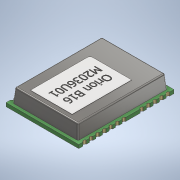
# Autodesk Inventor part: 03-0002
Saved by Autodesk Inventor 2021 (Build 250183000, 183)
## iProperties
Created: 2021-11-16
Part Number: 03-0002
Material: Stainless Steel
Document SubType Name: Modeling
Designer: Bradley
Density: 8 g/cm^3
Appearance: Semi-Polished
Author: Bradley
Autodesk Inventor part; units mm, degrees
ref_plane "YZ Plane" through (0, 0, 0) normal (1, 0, 0) x (0, 1, 0)
ref_plane "XZ Plane" through (0, 0, 0) normal (0, 1, 0) x (-1, 0, 0)
ref_plane "XY Plane" through (0, 0, 0) normal (0, 0, 1) x (1, 0, 0)
sketch "Sketch1" plane through (0, 0, 0) normal (0, 0, 1) x (1, 0, 0)
  line L0 (-6.1, -8) -> (6.1, -8)
  line L1 (6.1, -8) -> (6.1, 8)
  line L2 (6.1, 8) -> (-6.1, 8)
  line L3 (-6.1, 8) -> (-6.1, -8)
  line L4 (-6.1, -8) -> (6.1, 8) construction
  line L5 (6.1, -8) -> (-6.1, 8) construction
  point P0 (0, 0)
  dimension "d0" = 12.2
  dimension "d1" = 16
  constraints: 12 end point, 2 midpoint, 2 parallel, 1 horizontal, 1 perpendicular
  measures "d0" distance of L2.end L1.end
  measures "d1" distance of L1.end L0.end
extrude "Extrusion1" add sketch "Sketch1" along normal mid plane 0.6
sketch "Sketch2" plane through (0, 0, 0.3) normal (0, 0, 1) x (1, 0, 0)
  line L0 (6.1, -8) -> (6.1, 8) projected
  line L1 (6.1, 8) -> (-6.1, 8) projected
  line L2 (-6.1, 8) -> (-6.1, -8) projected
  line L3 (-6.1, -8) -> (6.1, -8) projected
  line L4 (-6.1, 8) -> (-6.1, -8) projected
  arc A0 (-6.1, 2.3) -> (-6.1, 2.9) centre (-6.2, 2.6) ccw
  line L5 (6.1, -8) -> (6.1, 8) projected
  arc A1 (6.1, 2.9) -> (6.1, 2.3) centre (6.2, 2.6) ccw
  arc A2 (-6.1, -7.3) -> (-6.1, -6.7) centre (-6.2, -7) ccw
  arc A3 (6.1, -6.7) -> (6.1, -7.3) centre (6.2, -7) ccw
  arc A4 (-6.1, 3.4) -> (-6.1, 4) centre (-6.2, 3.7) ccw
  arc A5 (6.1, 4) -> (6.1, 3.4) centre (6.2, 3.7) ccw
  arc A6 (-6.1, -6.2) -> (-6.1, -5.6) centre (-6.2, -5.9) ccw
  arc A7 (6.1, -5.6) -> (6.1, -6.2) centre (6.2, -5.9) ccw
  arc A8 (-6.1, 4.5) -> (-6.1, 5.1) centre (-6.2, 4.8) ccw
  arc A9 (6.1, 5.1) -> (6.1, 4.5) centre (6.2, 4.8) ccw
  arc A10 (-6.1, -5.1) -> (-6.1, -4.5) centre (-6.2, -4.8) ccw
  arc A11 (6.1, -4.5) -> (6.1, -5.1) centre (6.2, -4.8) ccw
  arc A12 (-6.1, 5.6) -> (-6.1, 6.2) centre (-6.2, 5.9) ccw
  arc A13 (6.1, 6.2) -> (6.1, 5.6) centre (6.2, 5.9) ccw
  arc A14 (-6.1, -4) -> (-6.1, -3.4) centre (-6.2, -3.7) ccw
  arc A15 (6.1, -3.4) -> (6.1, -4) centre (6.2, -3.7) ccw
  arc A16 (-6.1, 6.7) -> (-6.1, 7.3) centre (-6.2, 7) ccw
  arc A17 (6.1, 7.3) -> (6.1, 6.7) centre (6.2, 7) ccw
  arc A18 (-6.1, -2.9) -> (-6.1, -2.3) centre (-6.2, -2.6) ccw
  arc A19 (6.1, -2.3) -> (6.1, -2.9) centre (6.2, -2.6) ccw
  arc A20 (-6.1, 7.8) -> (-6.1, 8.4) centre (-6.2, 8.1) ccw
  arc A21 (6.1, 8.4) -> (6.1, 7.8) centre (6.2, 8.1) ccw
  arc A22 (-6.1, -1.8) -> (-6.1, -1.2) centre (-6.2, -1.5) ccw
  arc A23 (6.1, -1.2) -> (6.1, -1.8) centre (6.2, -1.5) ccw
  arc A24 (-6.1, 8.9) -> (-6.1, 9.5) centre (-6.2, 9.2) ccw
  arc A25 (6.1, 9.5) -> (6.1, 8.9) centre (6.2, 9.2) ccw
  arc A26 (-6.1, -0.7) -> (-6.1, -0.1) centre (-6.2, -0.4) ccw
  arc A27 (6.1, -0.1) -> (6.1, -0.7) centre (6.2, -0.4) ccw
  point P0 (0, 0)
  point P1 (-6.1, -5.1)
  point P2 (-6.1, -0.1)
  point P3 (-6.1, 2.9)
  point P4 (-6.1, 4)
  point P5 (6.1, 5.6)
  point P6 (6.1, 3.4)
  point P7 (6.1, 2.3)
  point P8 (6.1, -0.7)
  point P9 (6.1, -1.8)
  point P10 (6.1, -2.9)
  point P11 (6.1, -4)
  point P12 (6.1, -6.2)
  point P13 (6.1, -7.3)
  dimension "d4" = 1
  dimension "d5" = 0.6
  dimension "d6" = 0.1
  dimension "d7" = 0.1
  dimension "d10" = 1.1
  dimension "d15" = 3
  constraints: 74 vertical alignment, 56 point on circle, 28 centre point, 27 equal radius, 8 point on line, 2 horizontal alignment, 2 other
  measures "d4" distance from line of L3 A3.centre
  measures "d5" distance of A3.end A3.start
  measures "d10" distance of A0.start A4.start
  measures "d15" distance of A27.centre A1.centre
extrude "Extrusion2" cut sketch "Sketch2" against normal through all contours A3 L0 | L2 A2 | A7 L0 | L2 A6 | A11 L0 | L2 A10 | A15 L0 | L2 A14 | A19 L0 | L2 A18 | A23 L0 | L2 A22 | A27 L0 | L2 A26 | A1 L0 | L2 A0 | A5 L0 | L2 A4 | A9 L0 | L2 A8 | A13 L0 | L2 A12 | A17 L0 | L2 A16
sketch "Sketch3" plane through (0, 0, 0.3) normal (0, 0, 1) x (1, 0, 0)
  arc A0 (6.1, -4.5) -> (6.1, -5.1) centre (6.2, -4.8) ccw projected
  line L0 (6.1, -4.5) -> (6.1, -4) projected
  arc A1 (6.1, -3.4) -> (6.1, -4) centre (6.2, -3.7) ccw projected
  line L1 (6.1, -3.4) -> (6.1, -2.9) projected
  arc A2 (6.1, -2.3) -> (6.1, -2.9) centre (6.2, -2.6) ccw projected
  line L2 (6.1, -2.3) -> (6.1, -1.8) projected
  arc A3 (6.1, -1.2) -> (6.1, -1.8) centre (6.2, -1.5) ccw projected
  line L3 (6.1, -1.2) -> (6.1, -0.7) projected
  arc A4 (6.1, -0.1) -> (6.1, -0.7) centre (6.2, -0.4) ccw projected
  line L4 (6.1, -0.1) -> (6.1, 2.3) projected
  arc A5 (6.1, 2.9) -> (6.1, 2.3) centre (6.2, 2.6) ccw projected
  line L5 (6.1, 2.9) -> (6.1, 3.4) projected
  arc A6 (6.1, 4) -> (6.1, 3.4) centre (6.2, 3.7) ccw projected
  line L6 (6.1, 4) -> (6.1, 4.5) projected
  arc A7 (6.1, 5.1) -> (6.1, 4.5) centre (6.2, 4.8) ccw projected
  line L7 (6.1, 5.1) -> (6.1, 5.6) projected
  arc A8 (6.1, 6.2) -> (6.1, 5.6) centre (6.2, 5.9) ccw projected
  line L8 (6.1, 6.2) -> (6.1, 6.7) projected
  arc A9 (6.1, 7.3) -> (6.1, 6.7) centre (6.2, 7) ccw projected
  line L9 (6.1, 7.3) -> (6.1, 8) projected
  line L10 (6.1, 8) -> (-6.1, 8) projected
  line L11 (-6.1, 8) -> (-6.1, 7.3) projected
  arc A10 (-6.1, 6.7) -> (-6.1, 7.3) centre (-6.2, 7) ccw projected
  line L12 (-6.1, 6.7) -> (-6.1, 6.2) projected
  arc A11 (-6.1, 5.6) -> (-6.1, 6.2) centre (-6.2, 5.9) ccw projected
  line L13 (-6.1, 5.6) -> (-6.1, 5.1) projected
  arc A12 (-6.1, 4.5) -> (-6.1, 5.1) centre (-6.2, 4.8) ccw projected
  line L14 (-6.1, 4.5) -> (-6.1, 4) projected
  arc A13 (-6.1, 3.4) -> (-6.1, 4) centre (-6.2, 3.7) ccw projected
  line L15 (-6.1, 3.4) -> (-6.1, 2.9) projected
  arc A14 (-6.1, 2.3) -> (-6.1, 2.9) centre (-6.2, 2.6) ccw projected
  line L16 (-6.1, 2.3) -> (-6.1, -0.1) projected
  arc A15 (-6.1, -0.7) -> (-6.1, -0.1) centre (-6.2, -0.4) ccw projected
  line L17 (-6.1, -0.7) -> (-6.1, -1.2) projected
  arc A16 (-6.1, -1.8) -> (-6.1, -1.2) centre (-6.2, -1.5) ccw projected
  line L18 (-6.1, -1.8) -> (-6.1, -2.3) projected
  arc A17 (-6.1, -2.9) -> (-6.1, -2.3) centre (-6.2, -2.6) ccw projected
  line L19 (-6.1, -2.9) -> (-6.1, -3.4) projected
  arc A18 (-6.1, -4) -> (-6.1, -3.4) centre (-6.2, -3.7) ccw projected
  line L20 (-6.1, -4) -> (-6.1, -4.5) projected
  arc A19 (-6.1, -5.1) -> (-6.1, -4.5) centre (-6.2, -4.8) ccw projected
  line L21 (-6.1, -5.1) -> (-6.1, -5.6) projected
  arc A20 (-6.1, -6.2) -> (-6.1, -5.6) centre (-6.2, -5.9) ccw projected
  line L22 (-6.1, -6.2) -> (-6.1, -6.7) projected
  arc A21 (-6.1, -7.3) -> (-6.1, -6.7) centre (-6.2, -7) ccw projected
  line L23 (-6.1, -7.3) -> (-6.1, -8) projected
  line L24 (-6.1, -8) -> (6.1, -8) projected
  line L25 (6.1, -8) -> (6.1, -7.3) projected
  arc A22 (6.1, -6.7) -> (6.1, -7.3) centre (6.2, -7) ccw projected
  line L26 (6.1, -6.7) -> (6.1, -6.2) projected
  arc A23 (6.1, -5.6) -> (6.1, -6.2) centre (6.2, -5.9) ccw projected
  line L27 (6.1, -5.6) -> (6.1, -5.1) projected
  line L28 (-5.5, 7.5) -> (5.5, 7.5)
  line L29 (5.5, 7.5) -> (5.5, -7.5)
  line L30 (5.5, -7.5) -> (-5.5, -7.5)
  line L31 (-5.5, -7.5) -> (-5.5, 7.5)
  point P0 (0, 0)
  point P1 (0, 7.5)
  point P2 (-5.5, 0)
  dimension "d18" = 15
  dimension "d19" = 11
  constraints: 8 end point, 2 midpoint, 2 parallel, 1 horizontal, 1 horizontal alignment, 1 perpendicular, 1 vertical alignment
  measures "d18" distance of L30.end L28.start
  measures "d19" distance of L28.start L28.end
extrude "Extrusion3" add sketch "Sketch3" along normal blind 2.3 draft -5 contours L28 L29 L30 L31
fillet "Fillet1" radius 0.2 8 edges at (-5.2988, 0, 2.6) (-5.3994, 7.3994, 1.45) (-5.3994, -7.3994, 1.45) (0, 7.2988, 2.6) (5.3994, 7.3994, 1.45) (5.2988, 0, 2.6) (5.3994, -7.3994, 1.45) (0, -7.2988, 2.6)
sketch "Sketch4" plane through (0, 0, 2.6) normal (0, 0, 1) x (1, 0, 0)
  line L0 (3.5, 3.5) -> (-3, 3.5)
  line L1 (-3.5, 3) -> (-3.5, -6.5)
  line L2 (-3.5, -6.5) -> (3.5, -6.5)
  line L3 (3.5, -6.5) -> (3.5, 3.5)
  arc A0 (-3, 3.5) -> (-3.5, 3) centre (-3, 3) ccw
  point P0 (0, 0)
  point P1 (0, -6.5)
  dimension "d23" = 10
  dimension "d24" = 7
  dimension "d25" = 0.5
  dimension "d26" = 6.5
  constraints: 8 end point, 2 parallel, 2 point on circle, 2 tangent, 1 centre point, 1 horizontal, 1 midpoint, 1 perpendicular, 1 vertical alignment
  measures "d23" distance of L2.end L0.start
  measures "d24" distance of L1.end L2.end
  measures "d25" radius of A0
  measures "d26" distance from line of L2 point (0, 0)
emboss "Emboss1" sketch "Sketch4" operation add depth 0.05 direction (0, 0, -1)
sketch "Sketch5" plane through (-3.5, -6.5, 2.65) normal (0, 0, 1) x (1, 0, 0)
  line L0 (0.5, 10) -> (7, 10) construction
  line L1 (3.5, 10) -> (3.5, 0) construction
  line L2 (0, 0) -> (7, 0) construction
  spline S0 degree 2 poles (5.1072, 7.7624) (5.0241, 7.6915) (4.781, 7.6124) (4.625, 7.6124) knots 0 0 0 1 2 2 2
  spline S1 degree 2 poles (4.625, 7.6124) (4.4731, 7.6124) (4.2269, 7.6894) (4.1438, 7.7624) knots 0 0 0 1 2 2 2
  spline S2 degree 2 poles (4.1438, 7.7624) (4.0567, 7.8393) (3.9737, 8.0429) (3.9737, 8.1655) knots 0 0 0 1 2 2 2
  spline S3 degree 2 poles (3.9737, 8.1655) (3.9737, 8.2921) (4.0598, 8.4947) (4.1438, 8.5687) knots 0 0 0 1 2 2 2
  spline S4 degree 2 poles (4.1438, 8.5687) (4.2269, 8.6406) (4.471, 8.7176) (4.625, 8.7176) knots 0 0 0 1 2 2 2
  spline S5 degree 2 poles (4.625, 8.7176) (4.782, 8.7176) (5.0211, 8.6396) (5.1072, 8.5677) knots 0 0 0 1 2 2 2
  spline S6 degree 2 poles (5.1072, 8.5677) (5.1902, 8.4947) (5.2763, 8.2911) (5.2763, 8.1655) knots 0 0 0 1 2 2 2
  spline S7 degree 2 poles (5.2763, 8.1655) (5.2763, 8.0379) (5.1872, 7.8333) (5.1072, 7.7624) knots 0 0 0 1 2 2 2
  spline S8 degree 2 poles (4.625, 7.7857) (4.7486, 7.7857) (4.94, 7.8393) (5.0028, 7.888) knots 0 0 0 1 2 2 2
  spline S9 degree 2 poles (5.0028, 7.888) (5.0677, 7.9376) (5.1325, 8.0774) (5.1325, 8.1645) knots 0 0 0 1 2 2 2
  spline S10 degree 2 poles (5.1325, 8.1645) (5.1325, 8.2547) (5.0697, 8.3904) (5.0028, 8.4421) knots 0 0 0 1 2 2 2
  spline S11 degree 2 poles (5.0028, 8.4421) (4.939, 8.4917) (4.7466, 8.5444) (4.625, 8.5444) knots 0 0 0 1 2 2 2
  spline S12 degree 2 poles (4.625, 8.5444) (4.3788, 8.5444) (4.1175, 8.3377) (4.1175, 8.1645) knots 0 0 0 1 2 2 2
  spline S13 degree 2 poles (4.1175, 8.1645) (4.1175, 7.9913) (4.3788, 7.7857) (4.625, 7.7857) knots 0 0 0 1 2 2 2
  line L3 (4.7688, 6.9449) -> (4.7688, 6.953)
  spline S14 degree 2 poles (4.7688, 6.953) (4.7739, 6.9712) (4.7759, 7.0107) (4.7759, 7.0381) knots 0 0 0 1 2 2 2
  spline S15 degree 2 poles (4.7759, 7.0381) (4.7759, 7.1019) (4.7202, 7.2275) (4.6655, 7.2842) knots 0 0 0 1 2 2 2
  line L4 (4.6655, 7.2842) -> (4, 7.2842)
  line L5 (4, 7.2842) -> (4, 7.4423)
  line L6 (4, 7.4423) -> (4.938, 7.4423)
  line L7 (4.938, 7.4423) -> (4.938, 7.2842)
  line L8 (4.938, 7.2842) -> (4.7982, 7.2842)
  spline S16 degree 2 poles (4.7982, 7.2842) (4.8752, 7.1981) (4.938, 7.0695) (4.938, 7.0087) knots 0 0 0 1 2 2 2
  spline S17 degree 2 poles (4.938, 7.0087) (4.938, 6.9844) (4.936, 6.9601) (4.9329, 6.9449) knots 0 0 0 1 2 2 2
  line L9 (4.9329, 6.9449) -> (4.7688, 6.9449)
  line L10 (4, 6.6613) -> (4, 6.8193)
  line L11 (4, 6.8193) -> (4.938, 6.8193)
  line L12 (4.938, 6.8193) -> (4.938, 6.6613)
  line L13 (4.938, 6.6613) -> (4, 6.6613)
  line L14 (5.094, 6.6501) -> (5.094, 6.8294)
  line L15 (5.094, 6.8294) -> (5.2581, 6.8294)
  line L16 (5.2581, 6.8294) -> (5.2581, 6.6501)
  line L17 (5.2581, 6.6501) -> (5.094, 6.6501)
  spline S18 degree 2 poles (4.469, 5.6584) (4.232, 5.6584) (3.9737, 5.8863) (3.9737, 6.0768) knots 0 0 0 1 2 2 2
  spline S19 degree 2 poles (3.9737, 6.0768) (3.9737, 6.2723) (4.2401, 6.4962) (4.469, 6.4962) knots 0 0 0 1 2 2 2
  spline S20 degree 2 poles (4.469, 6.4962) (4.704, 6.4962) (4.9643, 6.2652) (4.9643, 6.0768) knots 0 0 0 1 2 2 2
  spline S21 degree 2 poles (4.9643, 6.0768) (4.9643, 5.8863) (4.705, 5.6584) (4.469, 5.6584) knots 0 0 0 1 2 2 2
  spline S22 degree 2 poles (4.469, 5.8215) (4.6513, 5.8215) (4.8286, 5.9542) (4.8286, 6.0768) knots 0 0 0 1 2 2 2
  spline S23 degree 2 poles (4.8286, 6.0768) (4.8286, 6.1994) (4.6513, 6.3331) (4.469, 6.3331) knots 0 0 0 1 2 2 2
  spline S24 degree 2 poles (4.469, 6.3331) (4.2917, 6.3331) (4.1094, 6.1994) (4.1094, 6.0768) knots 0 0 0 1 2 2 2
  spline S25 degree 2 poles (4.1094, 6.0768) (4.1094, 5.9552) (4.2887, 5.8215) (4.469, 5.8215) knots 0 0 0 1 2 2 2
  line L18 (4, 4.7599) -> (4, 4.9179)
  line L19 (4, 4.9179) -> (4.5348, 4.9179)
  spline S26 degree 2 poles (4.5348, 4.9179) (4.5997, 4.9179) (4.7111, 4.9301) (4.7445, 4.9483) knots 0 0 0 1 2 2 2
  spline S27 degree 2 poles (4.7445, 4.9483) (4.78, 4.9676) (4.8144, 5.0365) (4.8144, 5.0952) knots 0 0 0 1 2 2 2
  spline S28 degree 2 poles (4.8144, 5.0952) (4.8144, 5.154) (4.7516, 5.2786) (4.701, 5.3383) knots 0 0 0 1 2 2 2
  line L20 (4.701, 5.3383) -> (4, 5.3383)
  line L21 (4, 5.3383) -> (4, 5.4964)
  line L22 (4, 5.4964) -> (4.938, 5.4964)
  line L23 (4.938, 5.4964) -> (4.938, 5.3383)
  line L24 (4.938, 5.3383) -> (4.8337, 5.3383)
  spline S29 degree 2 poles (4.8337, 5.3383) (4.8975, 5.2674) (4.9643, 5.1307) (4.9643, 5.0537) knots 0 0 0 1 2 2 2
  spline S30 degree 2 poles (4.9643, 5.0537) (4.9643, 4.9159) (4.782, 4.7599) (4.6088, 4.7599) knots 0 0 0 1 2 2 2
  line L25 (4.6088, 4.7599) -> (4, 4.7599)
  spline S31 degree 2 poles (4.3839, 3.1412) (4.2907, 3.1412) (4.1479, 3.2121) (4.1013, 3.2709) knots 0 0 0 1 2 2 2
  spline S32 degree 2 poles (4.1013, 3.2709) (4.0466, 3.3418) (4, 3.5028) (4, 3.6305) knots 0 0 0 1 2 2 2
  line L26 (4, 3.6305) -> (4, 3.9891)
  line L27 (4, 3.9891) -> (5.25, 3.9891)
  line L28 (5.25, 3.9891) -> (5.25, 3.6578)
  spline S33 degree 2 poles (5.25, 3.6578) (5.25, 3.5241) (5.2328, 3.3904) (5.1994, 3.3296) knots 0 0 0 1 2 2 2
  spline S34 degree 2 poles (5.1994, 3.3296) (5.1639, 3.2618) (5.0474, 3.2) (4.9684, 3.2) knots 0 0 0 1 2 2 2
  spline S35 degree 2 poles (4.9684, 3.2) (4.8803, 3.2) (4.7405, 3.2932) (4.701, 3.3752) knots 0 0 0 1 2 2 2
  line L29 (4.701, 3.3752) -> (4.6949, 3.3752)
  spline S36 degree 2 poles (4.6949, 3.3752) (4.6645, 3.2638) (4.5034, 3.1412) (4.3839, 3.1412) knots 0 0 0 1 2 2 2
  spline S37 degree 2 poles (4.3768, 3.3144) (4.4477, 3.3144) (4.5389, 3.3549) (4.5713, 3.4157) knots 0 0 0 1 2 2 2
  spline S38 degree 2 poles (4.5713, 3.4157) (4.5916, 3.4552) (4.6037, 3.5484) (4.6037, 3.6345) knots 0 0 0 1 2 2 2
  line L30 (4.6037, 3.6345) -> (4.6037, 3.8229)
  line L31 (4.6037, 3.8229) -> (4.1418, 3.8229)
  line L32 (4.1418, 3.8229) -> (4.1418, 3.6882)
  spline S39 degree 2 poles (4.1418, 3.6882) (4.1418, 3.5788) (4.1621, 3.4532) (4.1945, 3.4046) knots 0 0 0 1 2 2 2
  spline S40 degree 2 poles (4.1945, 3.4046) (4.2279, 3.358) (4.311, 3.3144) (4.3768, 3.3144) knots 0 0 0 1 2 2 2
  spline S41 degree 2 poles (4.9451, 3.3732) (4.9897, 3.3732) (5.0565, 3.4036) (5.0758, 3.437) knots 0 0 0 1 2 2 2
  spline S42 degree 2 poles (5.0758, 3.437) (5.0981, 3.4775) (5.1082, 3.5758) (5.1082, 3.6639) knots 0 0 0 1 2 2 2
  line L33 (5.1082, 3.6639) -> (5.1082, 3.8229)
  line L34 (5.1082, 3.8229) -> (4.7425, 3.8229)
  line L35 (4.7425, 3.8229) -> (4.7425, 3.6345)
  spline S43 degree 2 poles (4.7425, 3.6345) (4.7425, 3.5565) (4.7587, 3.4826) (4.784, 3.4431) knots 0 0 0 1 2 2 2
  spline S44 degree 2 poles (4.784, 3.4431) (4.8083, 3.4046) (4.8863, 3.3732) (4.9451, 3.3732) knots 0 0 0 1 2 2 2
  line L36 (4, 2.3035) -> (4, 2.9133)
  line L37 (4, 2.9133) -> (4.1276, 2.9133)
  line L38 (4.1276, 2.9133) -> (4.1276, 2.6864)
  line L39 (4.1276, 2.6864) -> (4.9654, 2.6864)
  line L40 (4.9654, 2.6864) -> (4.9654, 2.9133)
  line L41 (4.9654, 2.9133) -> (5.0798, 2.9133)
  spline S45 degree 2 poles (5.0798, 2.9133) (5.0798, 2.7846) (5.1528, 2.6631) (5.2541, 2.655) knots 0 0 0 1 2 2 2
  line L42 (5.2541, 2.655) -> (5.2541, 2.5253)
  line L43 (5.2541, 2.5253) -> (4.1276, 2.5253)
  line L44 (4.1276, 2.5253) -> (4.1276, 2.3035)
  line L45 (4.1276, 2.3035) -> (4, 2.3035)
  spline S46 degree 2 poles (4.4052, 1.2834) (4.309, 1.2834) (4.1459, 1.3472) (4.0912, 1.4009) knots 0 0 0 1 2 2 2
  spline S47 degree 2 poles (4.0912, 1.4009) (4.0334, 1.4566) (3.9737, 1.5964) (3.9737, 1.6805) knots 0 0 0 1 2 2 2
  spline S48 degree 2 poles (3.9737, 1.6805) (3.9737, 1.7646) (4.0304, 1.9034) (4.0871, 1.956) knots 0 0 0 1 2 2 2
  spline S49 degree 2 poles (4.0871, 1.956) (4.155, 2.0209) (4.3829, 2.0938) (4.549, 2.0938) knots 0 0 0 1 2 2 2
  spline S50 degree 2 poles (4.549, 2.0938) (4.7121, 2.0938) (4.9745, 2.0269) (5.0717, 1.9571) knots 0 0 0 1 2 2 2
  spline S51 degree 2 poles (5.0717, 1.9571) (5.1669, 1.8892) (5.2733, 1.6744) (5.2733, 1.5336) knots 0 0 0 1 2 2 2
  spline S52 degree 2 poles (5.2733, 1.5336) (5.2733, 1.4921) (5.2652, 1.4192) (5.2561, 1.3918) knots 0 0 0 1 2 2 2
  line L46 (5.2561, 1.3918) -> (5.095, 1.3918)
  line L47 (5.095, 1.3918) -> (5.095, 1.3989)
  spline S53 degree 2 poles (5.095, 1.3989) (5.1072, 1.4222) (5.1284, 1.5073) (5.1284, 1.5559) knots 0 0 0 1 2 2 2
  spline S54 degree 2 poles (5.1284, 1.5559) (5.1284, 1.7119) (4.9177, 1.9034) (4.7111, 1.9216) knots 0 0 0 1 2 2 2
  spline S55 degree 2 poles (4.7111, 1.9216) (4.7526, 1.8618) (4.7982, 1.7362) (4.7982, 1.6613) knots 0 0 0 1 2 2 2
  spline S56 degree 2 poles (4.7982, 1.6613) (4.7982, 1.5883) (4.7688, 1.4789) (4.7243, 1.4192) knots 0 0 0 1 2 2 2
  spline S57 degree 2 poles (4.7243, 1.4192) (4.6726, 1.3503) (4.5126, 1.2834) (4.4052, 1.2834) knots 0 0 0 1 2 2 2
  spline S58 degree 2 poles (4.3981, 1.4536) (4.4751, 1.4536) (4.5794, 1.4941) (4.6159, 1.5387) knots 0 0 0 1 2 2 2
  spline S59 degree 2 poles (4.6159, 1.5387) (4.6422, 1.5721) (4.6594, 1.6552) (4.6594, 1.6987) knots 0 0 0 1 2 2 2
  spline S60 degree 2 poles (4.6594, 1.6987) (4.6594, 1.7575) (4.624, 1.8679) (4.5906, 1.9216) knots 0 0 0 1 2 2 2
  spline S61 degree 2 poles (4.5906, 1.9216) (4.5723, 1.9226) (4.5379, 1.9246) (4.5115, 1.9246) knots 0 0 0 1 2 2 2
  spline S62 degree 2 poles (4.5115, 1.9246) (4.3819, 1.9246) (4.2229, 1.874) (4.1813, 1.8355) knots 0 0 0 1 2 2 2
  spline S63 degree 2 poles (4.1813, 1.8355) (4.1418, 1.8) (4.1104, 1.7231) (4.1104, 1.6795) knots 0 0 0 1 2 2 2
  spline S64 degree 2 poles (4.1104, 1.6795) (4.1104, 1.5782) (4.2543, 1.4536) (4.3981, 1.4536) knots 0 0 0 1 2 2 2
  line L48 (1.9358, 7.8419) -> (1.9358, 8.008)
  line L49 (1.9358, 8.008) -> (3.0126, 8.008)
  line L50 (3.0126, 8.008) -> (2.2802, 8.3342)
  line L51 (2.2802, 8.3342) -> (2.2802, 8.4355)
  line L52 (2.2802, 8.4355) -> (3.0126, 8.7586)
  line L53 (3.0126, 8.7586) -> (1.9358, 8.7586)
  line L54 (1.9358, 8.7586) -> (1.9358, 8.9136)
  line L55 (1.9358, 8.9136) -> (3.1858, 8.9136)
  line L56 (3.1858, 8.9136) -> (3.1858, 8.6867)
  line L57 (3.1858, 8.6867) -> (2.4899, 8.3747)
  line L58 (2.4899, 8.3747) -> (3.1858, 8.0728)
  line L59 (3.1858, 8.0728) -> (3.1858, 7.8419)
  line L60 (3.1858, 7.8419) -> (1.9358, 7.8419)
  line L61 (1.9358, 6.8532) -> (1.9358, 7.6241)
  line L62 (1.9358, 7.6241) -> (2.1131, 7.6241)
  spline S65 degree 2 poles (2.1131, 7.6241) (2.1911, 7.541) (2.3359, 7.3931) (2.4139, 7.3222) knots 0 0 0 1 2 2 2
  spline S66 degree 2 poles (2.4139, 7.3222) (2.5709, 7.1794) (2.7593, 7.0751) (2.8596, 7.0751) knots 0 0 0 1 2 2 2
  spline S67 degree 2 poles (2.8596, 7.0751) (2.9123, 7.0751) (2.9913, 7.1075) (3.0166, 7.1369) knots 0 0 0 1 2 2 2
  spline S68 degree 2 poles (3.0166, 7.1369) (3.042, 7.1662) (3.0673, 7.2432) (3.0673, 7.2898) knots 0 0 0 1 2 2 2
  spline S69 degree 2 poles (3.0673, 7.2898) (3.0673, 7.3344) (3.045, 7.4255) (3.0278, 7.4671) knots 0 0 0 1 2 2 2
  spline S70 degree 2 poles (3.0278, 7.4671) (3.0136, 7.5025) (2.9731, 7.5684) (2.9589, 7.5886) knots 0 0 0 1 2 2 2
  line L63 (2.9589, 7.5886) -> (2.9589, 7.5978)
  line L64 (2.9589, 7.5978) -> (3.1372, 7.5978)
  spline S71 degree 2 poles (3.1372, 7.5978) (3.1625, 7.5461) (3.2121, 7.3607) (3.2121, 7.2777) knots 0 0 0 1 2 2 2
  spline S72 degree 2 poles (3.2121, 7.2777) (3.2121, 7.1024) (3.0268, 6.9049) (2.8687, 6.9049) knots 0 0 0 1 2 2 2
  spline S73 degree 2 poles (2.8687, 6.9049) (2.7948, 6.9049) (2.6712, 6.9393) (2.6185, 6.9697) knots 0 0 0 1 2 2 2
  spline S74 degree 2 poles (2.6185, 6.9697) (2.5638, 7.0001) (2.4565, 7.0882) (2.4048, 7.1369) knots 0 0 0 1 2 2 2
  spline S75 degree 2 poles (2.4048, 7.1369) (2.3187, 7.2159) (2.1343, 7.4093) (2.0807, 7.4671) knots 0 0 0 1 2 2 2
  line L65 (2.0807, 7.4671) -> (2.0807, 6.8532)
  line L66 (2.0807, 6.8532) -> (1.9358, 6.8532)
  spline S76 degree 2 poles (2.5608, 5.9081) (2.2245, 5.9081) (1.9095, 6.1036) (1.9095, 6.3072) knots 0 0 0 1 2 2 2
  spline S77 degree 2 poles (1.9095, 6.3072) (1.9095, 6.5139) (2.2306, 6.7074) (2.5598, 6.7074) knots 0 0 0 1 2 2 2
  spline S78 degree 2 poles (2.5598, 6.7074) (2.8981, 6.7074) (3.2111, 6.5119) (3.2111, 6.3072) knots 0 0 0 1 2 2 2
  spline S79 degree 2 poles (3.2111, 6.3072) (3.2111, 6.1016) (2.887, 5.9081) (2.5608, 5.9081) knots 0 0 0 1 2 2 2
  spline S80 degree 2 poles (2.1799, 6.1229) (2.2417, 6.0986) (2.4322, 6.0783) (2.5608, 6.0783) knots 0 0 0 1 2 2 2
  spline S81 degree 2 poles (2.5608, 6.0783) (2.6894, 6.0783) (2.8789, 6.0986) (2.9427, 6.1239) knots 0 0 0 1 2 2 2
  spline S82 degree 2 poles (2.9427, 6.1239) (3.0065, 6.1492) (3.0723, 6.2373) (3.0723, 6.3072) knots 0 0 0 1 2 2 2
  spline S83 degree 2 poles (3.0723, 6.3072) (3.0723, 6.3771) (3.0065, 6.4673) (2.9407, 6.4936) knots 0 0 0 1 2 2 2
  spline S84 degree 2 poles (2.9407, 6.4936) (2.8768, 6.5189) (2.6824, 6.5372) (2.5598, 6.5372) knots 0 0 0 1 2 2 2
  spline S85 degree 2 poles (2.5598, 6.5372) (2.4281, 6.5372) (2.2518, 6.521) (2.183, 6.4946) knots 0 0 0 1 2 2 2
  spline S86 degree 2 poles (2.183, 6.4946) (2.1181, 6.4703) (2.0482, 6.3802) (2.0482, 6.3072) knots 0 0 0 1 2 2 2
  spline S87 degree 2 poles (2.0482, 6.3072) (2.0482, 6.2384) (2.1141, 6.1482) (2.1799, 6.1229) knots 0 0 0 1 2 2 2
  spline S88 degree 2 poles (3.0673, 5.4108) (3.0673, 5.4563) (3.045, 5.5465) (3.0278, 5.5901) knots 0 0 0 1 2 2 2
  spline S89 degree 2 poles (3.0278, 5.5901) (3.0106, 5.6306) (2.9741, 5.6903) (2.9579, 5.7136) knots 0 0 0 1 2 2 2
  line L67 (2.9579, 5.7136) -> (2.9579, 5.7238)
  line L68 (2.9579, 5.7238) -> (3.1352, 5.7238)
  spline S90 degree 2 poles (3.1352, 5.7238) (3.1645, 5.6691) (3.2121, 5.4817) (3.2121, 5.3976) knots 0 0 0 1 2 2 2
  spline S91 degree 2 poles (3.2121, 5.3976) (3.2121, 5.3125) (3.1777, 5.1859) (3.1412, 5.1342) knots 0 0 0 1 2 2 2
  spline S92 degree 2 poles (3.1412, 5.1342) (3.1017, 5.0795) (2.9873, 5.0228) (2.9103, 5.0228) knots 0 0 0 1 2 2 2
  spline S93 degree 2 poles (2.9103, 5.0228) (2.807, 5.0228) (2.651, 5.1585) (2.6307, 5.2537) knots 0 0 0 1 2 2 2
  line L69 (2.6307, 5.2537) -> (2.6185, 5.2537)
  spline S94 degree 2 poles (2.6185, 5.2537) (2.6104, 5.2142) (2.574, 5.1241) (2.5375, 5.0856) knots 0 0 0 1 2 2 2
  spline S95 degree 2 poles (2.5375, 5.0856) (2.502, 5.0471) (2.3886, 4.9985) (2.3065, 4.9985) knots 0 0 0 1 2 2 2
  spline S96 degree 2 poles (2.3065, 4.9985) (2.2225, 4.9985) (2.0796, 5.0562) (2.0249, 5.1089) knots 0 0 0 1 2 2 2
  spline S97 degree 2 poles (2.0249, 5.1089) (1.9682, 5.1636) (1.9095, 5.3186) (1.9095, 5.4168) knots 0 0 0 1 2 2 2
  spline S98 degree 2 poles (1.9095, 5.4168) (1.9095, 5.511) (1.955, 5.6954) (1.9864, 5.7582) knots 0 0 0 1 2 2 2
  line L70 (1.9864, 5.7582) -> (2.1637, 5.7582)
  line L71 (2.1637, 5.7582) -> (2.1637, 5.746)
  spline S99 degree 2 poles (2.1637, 5.746) (2.1252, 5.6934) (2.0543, 5.5151) (2.0543, 5.427) knots 0 0 0 1 2 2 2
  spline S100 degree 2 poles (2.0543, 5.427) (2.0543, 5.3753) (2.0867, 5.272) (2.1242, 5.2375) knots 0 0 0 1 2 2 2
  spline S101 degree 2 poles (2.1242, 5.2375) (2.1617, 5.2041) (2.2508, 5.1687) (2.3187, 5.1687) knots 0 0 0 1 2 2 2
  spline S102 degree 2 poles (2.3187, 5.1687) (2.3866, 5.1687) (2.4747, 5.2082) (2.5, 5.2436) knots 0 0 0 1 2 2 2
  spline S103 degree 2 poles (2.5, 5.2436) (2.5253, 5.2791) (2.5446, 5.3753) (2.5446, 5.432) knots 0 0 0 1 2 2 2
  line L72 (2.5446, 5.432) -> (2.5446, 5.5029)
  line L73 (2.5446, 5.5029) -> (2.6834, 5.5029)
  line L74 (2.6834, 5.5029) -> (2.6834, 5.4472)
  spline S104 degree 2 poles (2.6834, 5.4472) (2.6834, 5.3348) (2.7907, 5.193) (2.8931, 5.193) knots 0 0 0 1 2 2 2
  spline S105 degree 2 poles (2.8931, 5.193) (2.9407, 5.193) (3.0085, 5.2294) (3.0288, 5.2588) knots 0 0 0 1 2 2 2
  spline S106 degree 2 poles (3.0288, 5.2588) (3.0501, 5.2902) (3.0673, 5.3672) (3.0673, 5.4108) knots 0 0 0 1 2 2 2
  spline S107 degree 2 poles (2.341, 4.02) (2.2448, 4.02) (2.0817, 4.0838) (2.027, 4.1375) knots 0 0 0 1 2 2 2
  spline S108 degree 2 poles (2.027, 4.1375) (1.9692, 4.1932) (1.9095, 4.333) (1.9095, 4.417) knots 0 0 0 1 2 2 2
  spline S109 degree 2 poles (1.9095, 4.417) (1.9095, 4.5011) (1.9662, 4.6399) (2.0229, 4.6926) knots 0 0 0 1 2 2 2
  spline S110 degree 2 poles (2.0229, 4.6926) (2.0908, 4.7574) (2.3187, 4.8303) (2.4848, 4.8303) knots 0 0 0 1 2 2 2
  spline S111 degree 2 poles (2.4848, 4.8303) (2.6479, 4.8303) (2.9103, 4.7635) (3.0075, 4.6936) knots 0 0 0 1 2 2 2
  spline S112 degree 2 poles (3.0075, 4.6936) (3.1027, 4.6257) (3.2091, 4.411) (3.2091, 4.2702) knots 0 0 0 1 2 2 2
  spline S113 degree 2 poles (3.2091, 4.2702) (3.2091, 4.2286) (3.201, 4.1557) (3.1919, 4.1283) knots 0 0 0 1 2 2 2
  line L75 (3.1919, 4.1283) -> (3.0308, 4.1283)
  line L76 (3.0308, 4.1283) -> (3.0308, 4.1354)
  spline S114 degree 2 poles (3.0308, 4.1354) (3.043, 4.1587) (3.0642, 4.2438) (3.0642, 4.2924) knots 0 0 0 1 2 2 2
  spline S115 degree 2 poles (3.0642, 4.2924) (3.0642, 4.4484) (2.8535, 4.6399) (2.6469, 4.6581) knots 0 0 0 1 2 2 2
  spline S116 degree 2 poles (2.6469, 4.6581) (2.6884, 4.5984) (2.734, 4.4728) (2.734, 4.3978) knots 0 0 0 1 2 2 2
  spline S117 degree 2 poles (2.734, 4.3978) (2.734, 4.3249) (2.7046, 4.2155) (2.6601, 4.1557) knots 0 0 0 1 2 2 2
  spline S118 degree 2 poles (2.6601, 4.1557) (2.6084, 4.0868) (2.4484, 4.02) (2.341, 4.02) knots 0 0 0 1 2 2 2
  spline S119 degree 2 poles (2.3339, 4.1901) (2.4109, 4.1901) (2.5152, 4.2307) (2.5517, 4.2752) knots 0 0 0 1 2 2 2
  spline S120 degree 2 poles (2.5517, 4.2752) (2.578, 4.3087) (2.5952, 4.3917) (2.5952, 4.4353) knots 0 0 0 1 2 2 2
  spline S121 degree 2 poles (2.5952, 4.4353) (2.5952, 4.494) (2.5598, 4.6044) (2.5264, 4.6581) knots 0 0 0 1 2 2 2
  spline S122 degree 2 poles (2.5264, 4.6581) (2.5081, 4.6591) (2.4737, 4.6612) (2.4473, 4.6612) knots 0 0 0 1 2 2 2
  spline S123 degree 2 poles (2.4473, 4.6612) (2.3177, 4.6612) (2.1587, 4.6105) (2.1171, 4.572) knots 0 0 0 1 2 2 2
  spline S124 degree 2 poles (2.1171, 4.572) (2.0776, 4.5366) (2.0462, 4.4596) (2.0462, 4.416) knots 0 0 0 1 2 2 2
  spline S125 degree 2 poles (2.0462, 4.416) (2.0462, 4.3147) (2.1901, 4.1901) (2.3339, 4.1901) knots 0 0 0 1 2 2 2
  spline S126 degree 2 poles (1.9095, 3.4) (1.9095, 3.5104) (1.9672, 3.6745) (2.0249, 3.7323) knots 0 0 0 1 2 2 2
  spline S127 degree 2 poles (2.0249, 3.7323) (2.0898, 3.7981) (2.2721, 3.8518) (2.4058, 3.8518) knots 0 0 0 1 2 2 2
  line L77 (2.4058, 3.8518) -> (3.1858, 3.8518)
  line L78 (3.1858, 3.8518) -> (3.1858, 3.6857)
  line L79 (3.1858, 3.6857) -> (2.4058, 3.6857)
  spline S128 degree 2 poles (2.4058, 3.6857) (2.3187, 3.6857) (2.2012, 3.6634) (2.1536, 3.632) knots 0 0 0 1 2 2 2
  spline S129 degree 2 poles (2.1536, 3.632) (2.1029, 3.5986) (2.0513, 3.4831) (2.0513, 3.4) knots 0 0 0 1 2 2 2
  spline S130 degree 2 poles (2.0513, 3.4) (2.0513, 3.322) (2.1029, 3.2005) (2.1536, 3.167) knots 0 0 0 1 2 2 2
  spline S131 degree 2 poles (2.1536, 3.167) (2.2012, 3.1356) (2.3177, 3.1134) (2.4018, 3.1134) knots 0 0 0 1 2 2 2
  line L80 (2.4018, 3.1134) -> (3.1858, 3.1134)
  line L81 (3.1858, 3.1134) -> (3.1858, 2.9472)
  line L82 (3.1858, 2.9472) -> (2.4058, 2.9472)
  spline S132 degree 2 poles (2.4058, 2.9472) (2.2751, 2.9472) (2.0888, 2.9999) (2.0249, 3.0668) knots 0 0 0 1 2 2 2
  spline S133 degree 2 poles (2.0249, 3.0668) (1.9662, 3.1265) (1.9095, 3.2845) (1.9095, 3.4) knots 0 0 0 1 2 2 2
  spline S134 degree 2 poles (2.5608, 1.9667) (2.2245, 1.9667) (1.9095, 2.1622) (1.9095, 2.3658) knots 0 0 0 1 2 2 2
  spline S135 degree 2 poles (1.9095, 2.3658) (1.9095, 2.5724) (2.2306, 2.7659) (2.5598, 2.7659) knots 0 0 0 1 2 2 2
  spline S136 degree 2 poles (2.5598, 2.7659) (2.8981, 2.7659) (3.2111, 2.5704) (3.2111, 2.3658) knots 0 0 0 1 2 2 2
  spline S137 degree 2 poles (3.2111, 2.3658) (3.2111, 2.1601) (2.887, 1.9667) (2.5608, 1.9667) knots 0 0 0 1 2 2 2
  spline S138 degree 2 poles (2.1799, 2.1814) (2.2417, 2.1571) (2.4322, 2.1369) (2.5608, 2.1369) knots 0 0 0 1 2 2 2
  spline S139 degree 2 poles (2.5608, 2.1369) (2.6894, 2.1369) (2.8789, 2.1571) (2.9427, 2.1824) knots 0 0 0 1 2 2 2
  spline S140 degree 2 poles (2.9427, 2.1824) (3.0065, 2.2078) (3.0723, 2.2959) (3.0723, 2.3658) knots 0 0 0 1 2 2 2
  spline S141 degree 2 poles (3.0723, 2.3658) (3.0723, 2.4357) (3.0065, 2.5258) (2.9407, 2.5522) knots 0 0 0 1 2 2 2
  spline S142 degree 2 poles (2.9407, 2.5522) (2.8768, 2.5775) (2.6824, 2.5957) (2.5598, 2.5957) knots 0 0 0 1 2 2 2
  spline S143 degree 2 poles (2.5598, 2.5957) (2.4281, 2.5957) (2.2518, 2.5795) (2.183, 2.5532) knots 0 0 0 1 2 2 2
  spline S144 degree 2 poles (2.183, 2.5532) (2.1181, 2.5289) (2.0482, 2.4387) (2.0482, 2.3658) knots 0 0 0 1 2 2 2
  spline S145 degree 2 poles (2.0482, 2.3658) (2.0482, 2.2969) (2.1141, 2.2067) (2.1799, 2.1814) knots 0 0 0 1 2 2 2
  line L83 (1.9358, 1.0986) -> (1.9358, 1.7084)
  line L84 (1.9358, 1.7084) -> (2.0634, 1.7084)
  line L85 (2.0634, 1.7084) -> (2.0634, 1.4815)
  line L86 (2.0634, 1.4815) -> (2.9012, 1.4815)
  line L87 (2.9012, 1.4815) -> (2.9012, 1.7084)
  line L88 (2.9012, 1.7084) -> (3.0156, 1.7084)
  spline S146 degree 2 poles (3.0156, 1.7084) (3.0156, 1.5797) (3.0886, 1.4582) (3.1899, 1.4501) knots 0 0 0 1 2 2 2
  line L89 (3.1899, 1.4501) -> (3.1899, 1.3204)
  line L90 (3.1899, 1.3204) -> (2.0634, 1.3204)
  line L91 (2.0634, 1.3204) -> (2.0634, 1.0986)
  line L92 (2.0634, 1.0986) -> (1.9358, 1.0986)
  point P0 (3.5, 6.5)
  constraints: 2 end point, 2 vertical, 1 midpoint, 1 point on line
emboss "Emboss2" sketch "Sketch5" operation add depth 0.005 direction (0, 0, -1)
equation "\"d7\" = d6"
body "Solid1"
